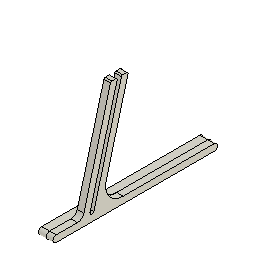
LCA 2021 Badge Stand v2 (Autodesk Fusion 360 design; units mm, degrees)
Autodesk Fusion 360 part; units mm, degrees
note: some values were not read from the file. Set by a fixed rule: which sketch regions a step uses.
sketch "Sketch1" plane through (0, 0, 0) normal (1, 0, 0) x (0, 1, 0)
  circle A0 centre (-67.573, 26.6271) radius 2.5
  line L0 (-67.573, 29.1271) -> (52.427, 29.1271)
  line L1 (52.427, 29.1271) -> (52.427, 24.1271)
  line L2 (52.427, 24.1271) -> (-67.573, 24.1271)
  line L3 (-67.573, 24.1271) -> (-67.573, 29.1271)
  circle A1 centre (52.427, 26.6271) radius 2.5
  line L4 (-47.573, 29.1271) -> (-47.573, 44.2726) construction
  line L5 (-47.573, 29.1271) -> (-26.3356, 108.3859)
  line L6 (-25.3697, 109.1271) -> (-22.2639, 109.1271)
  line L7 (-21.298, 107.8682) -> (-42.3966, 29.1271)
  line L8 (-39.2908, 29.1271) -> (-18.0534, 108.3859)
  line L9 (-13.0157, 107.8682) -> (-34.1144, 29.1271)
  line L10 (-17.0875, 109.1271) -> (-13.9817, 109.1271)
  arc A2 (-25.3697, 109.1271) -> (-26.3356, 108.3859) centre (-25.3697, 108.1271) ccw
  arc A3 (-21.298, 107.8682) -> (-22.2639, 109.1271) centre (-22.2639, 108.1271) ccw
  arc A4 (-17.0875, 109.1271) -> (-18.0534, 108.3859) centre (-17.0875, 108.1271) ccw
  arc A5 (-13.0157, 107.8682) -> (-13.9817, 109.1271) centre (-13.9817, 108.1271) ccw
  dimension "d6" = 5
  dimension "d7" = 120
  dimension "d8" = 5
  dimension "d9" = 20
  dimension "d10" = 3
  dimension "d11" = 5
  dimension "d12" = 5
  dimension "d13" = 75
  dimension "d16" = 1
  dimension "d17" = 1
  dimension "d18" = 1
  dimension "d19" = 1
  dimension "d20" = 80
  constraint horizontal L0
  constraint vertical L1
  constraint horizontal L2
  constraint vertical L3
  constraint coincident A0.centre L3
  constraint tangent A0 L0
  constraint tangent A0 L2
  constraint midpoint L1 A1.centre
  constraint coincident L0 L4.start
  constraint perpendicular L0 L4
  constraint perpendicular L4 L6
  constraint parallel L5 L7
  constraint coincident L0 L7.end
  constraint parallel L8 L9
  constraint coincident L0 L8.start
  constraint coincident L0 L9.end
  constraint collinear L6 L10
  constraint tangent L5 A2
  constraint tangent L6 A2
  constraint tangent L6 A3
  constraint tangent L7 A3
  constraint tangent L8 A4
  constraint tangent L10 A4
  constraint tangent L9 A5
  constraint tangent L10 A5
  measures "d6" diameter of A0
  measures "d7" distance of L0.start L1
  measures "d8" diameter of A1
  measures "d9" distance of L0.start L4
  measures "d10" distance of L7 L8
  measures "d11" distance of L5 L7
  measures "d12" distance of L8 L9
  measures "d13" angle of L0 L7
  measures "d16" radius of A2
  measures "d17" radius of A3
  measures "d18" radius of A4
  measures "d19" radius of A5
  measures "d20" distance of L0 L6
extrude "Extrude1" add sketch "Sketch1" along normal blind 5 makes body 1
fillet "FrontFillet" radius 5 1 edges at (2.5, -47.573, 29.1271) on bodies 1
fillet "RearArmFillet" radius 13.3333 1 edges at (2.5, -34.1144, 29.1271) on bodies 1
extrude "AddBaseThickener" add sketch "Sketch1" against normal blind 6 separate body contours A0 L3 | A0 L0 L2 A1 | A0 L3 | L1 A1 | L1 A1 makes body 2
copy_body "CutPasteBodies2" bodies 1 2 removing the originals makes body 3 makes body 4 in component "Component"
fillet "Fillet1" radius 1.5 1 edges at (2.5, -42.3966, 29.1271) on bodies 3 in component "Component"
fillet "Fillet2" radius 1.5 1 edges at (2.5, -39.2908, 29.1271) on bodies 3 in component "Component"
component "Component" placed x (1, 0, 0) y (0, 1, 0) z (0, 0, 1) at (0, 0, 0)
equation "boardthickness = 3 mm"
equation "fillet = 1 mm"
equation "basethickness = 5 mm"
equation "baselength = 120 mm"
equation "base_setback = 20 mm"
equation "d6 = basethickness"
equation "d7 = baselength"
equation "d8 = d6"
equation "d9 = base_setback"
equation "d10 = boardthickness"
equation "d11 = basethickness"
equation "d12 = d11"
equation "d13 = board_angle"
equation "board_angle = 75 deg"
equation "d16 = fillet"
equation "d17 = fillet"
equation "d20 = holderheight"
equation "holderheight = 80 mm"
equation "d25 = basethickness"
equation "d27 = holderheight / 6"
equation "d28 = -thickener"
equation "thickener = 6 mm"
equation "d32 = boardthickness / 2"
equation "d34 = boardthickness / 2"
named bodies: "MainBit", "Thicker_Base"
